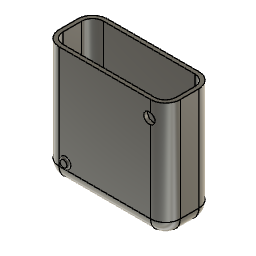
mucon_v2.6 (Autodesk Fusion 360 design; units mm, degrees)
Autodesk Fusion 360 part; units mm, degrees
sketch "スケッチ1" plane through (0, 0, 0) normal (0, 0, 1) x (1, 0, 0)
  line L0 (12.3, -4.9) -> (-12.3, -4.9)
  line L1 (-12.3, -4.9) -> (-12.3, 4.9)
  line L2 (-12.3, 4.9) -> (12.3, 4.9)
  line L3 (12.3, 4.9) -> (12.3, -4.9)
  line L4 (12.3, -4.9) -> (-12.3, 4.9) construction
  line L5 (-12.3, -4.9) -> (12.3, 4.9) construction
  dimension "d1" = 24.6
  dimension "d2" = 9.8
  constraint horizontal L0
  constraint perpendicular L0 L1
  constraint parallel L0 L2
  constraint parallel L1 L3
  constraint coincident L4 origin
  constraint coincident L5 origin
  measures "d1" distance of L1.end L2.end
  measures "d2" distance of L0.end L1.end
extrude "押し出し1" add sketch "スケッチ1" along normal blind 24
fillet "フィレット2" radius 3 8 edges at (0, -4.9, 0) (12.3, 0, 0) (0, 4.9, 0) (-12.3, 0, 0) (12.3, -4.9, 12) (-12.3, -4.9, 12) (-12.3, 4.9, 12) (12.3, 4.9, 12)
shell "シェル2" thickness 0.8 removed faces 1 at (3.1, -1.6333, 24)
ref_plane "作業平面3" through (0, -4.9, 0) normal (0, 1, 0) x (0, 0, 1)
sketch "スケッチ2" plane through (0, -4.9, 0) normal (0, 1, 0) x (1, 0, 0)
  circle A0 centre (9, -20.6) radius 1.1
  line L0 (8.5, -0.6) -> (-8.5, -0.6)
  line L1 (-11.5, -3.6) -> (-11.5, -19.6)
  line L2 (-7.5, -23.6) -> (9, -23.6)
  line L3 (11.5, -21.1) -> (11.5, -3.6)
  line L4 (11.5, -0.6) -> (-11.5, -23.6) construction
  line L5 (-11.5, -0.6) -> (11.5, -23.6) construction
  arc A1 (-11.5, -19.6) -> (-7.5, -23.6) centre (-7.5, -19.6) ccw
  arc A2 (9, -23.6) -> (11.5, -21.1) centre (9, -21.1) ccw
  circle A3 centre (9, -21.1) radius 1.1
  arc A4 (11.5, -3.6) -> (8.5, -0.6) centre (8.5, -3.6) ccw
  arc A5 (-8.5, -0.6) -> (-11.5, -3.6) centre (-8.5, -3.6) ccw
  circle A6 centre (8, -12.1) radius 1.1
  circle A7 centre (8, -4.25) radius 1.1
  circle A8 centre (-8, -12.1) radius 1.1
  circle A9 centre (-8, -4.25) radius 1.1
  circle A10 centre (-8, -19.95) radius 1.1
  point P0 (0, -12.1)
  dimension "d19" = 2.2
  dimension "d22" = 23
  dimension "d23" = 23
  dimension "d24" = 4
  dimension "d25" = 2.5
  dimension "d26" = 2.2
  dimension "d27" = 3
  dimension "d28" = 3
  dimension "d30" = 2.2
  dimension "d31" = 2.2
  dimension "d32" = 2.2
  dimension "d33" = 2.2
  dimension "d34" = 2.2
  constraint horizontal L0
  constraint perpendicular L0 L1
  constraint parallel L0 L2
  constraint parallel L1 L3
  constraint coincident L4 P0
  constraint coincident L5 P0
  constraint coincident L4.end L2
  constraint coincident L4.end L1
  constraint tangent L2 A1
  constraint tangent L1 A1
  constraint coincident L5.end L2
  constraint coincident L5.end L3
  constraint tangent L2 A2
  constraint tangent L3 A2
  constraint coincident L4.start L3
  constraint coincident L4.start L0
  constraint tangent L3 A4
  constraint tangent L0 A4
  constraint coincident L5.start L1
  constraint coincident L5.start L0
  constraint tangent L1 A5
  constraint tangent L0 A5
  measures "d19" diameter of A0
  measures "d22" distance of L4.end L5.end
  measures "d23" distance of L5.start L4.end
  measures "d24" radius of A1
  measures "d25" radius of A2
  measures "d26" diameter of A3
  measures "d27" radius of A4
  measures "d28" radius of A5
  measures "d30" diameter of A6
  measures "d31" diameter of A7
  measures "d32" diameter of A8
  measures "d33" diameter of A9
  measures "d34" diameter of A10
extrude "押し出し3" cut sketch "スケッチ2" along normal blind 1.5 contours A0 A3 | A0 A3 picked at (9.093, -19.8394) picked at (9.0545, -21.1293)
extrude "押し出し4" add sketch "スケッチ2" against normal blind 0.4 contours A9
fillet "フィレット3" radius 0.4 1 edges at (-9.0256, -5.3, 3.8522)
